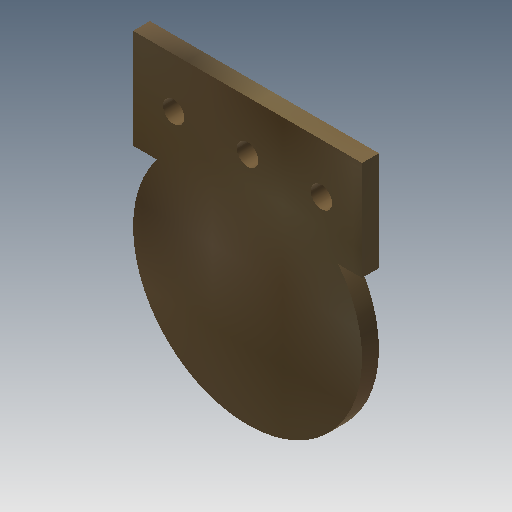
# Autodesk Inventor part: Part3_panel pot
Saved by Autodesk Inventor 2020 (Build 240168000, 168)
## iProperties
Created: 2016-08-22
Part Number: Part3_panel pot
Material: Generic
Document SubType Name: Modeling
Designer: Tom
Density: 1 g/cm^3
Appearance: Default
Author: Tom
Autodesk Inventor part; units mm, degrees
ref_plane "YZ Plane" through (0, 0, 0) normal (1, 0, 0) x (0, 1, 0)
ref_plane "XZ Plane" through (0, 0, 0) normal (0, 1, 0) x (-1, 0, 0)
ref_plane "XY Plane" through (0, 0, 0) normal (0, 0, 1) x (1, 0, 0)
sketch "Sketch1" plane through (0, 0, 0) normal (0, 0, 1) x (1, 0, 0)
  arc A0 (-6.1315, 4.735) -> (6.1315, 4.735) centre (0, 0) ccw
  line L0 (0, 0) -> (13.0157, 0) construction
  line L1 (7.747, 4.735) -> (7.747, 11.466)
  line L2 (7.747, 11.466) -> (-7.747, 11.466)
  line L3 (-7.747, 11.466) -> (-7.747, 4.735)
  line L4 (-7.747, 4.735) -> (-6.1315, 4.735)
  line L5 (6.1315, 4.735) -> (7.747, 4.735)
  dimension "d0" = 15.494
  dimension "d1" = 6.731
  dimension "d2" = 15.494
  dimension "d3" = 7.747
  constraints: 12 end point, 3 horizontal, 3 parallel, 2 perpendicular, 2 point on circle, 1 centre point, 1 coincident
  measures "d0" diameter of A0
  measures "d1" distance of L2.end L3.end
  measures "d2" distance of L1.end L2.end
  measures "d3" distance from line of L1 point (0, 0)
extrude "Extrusion1" add sketch "Sketch1" along normal blind 1.143
sketch "Sketch2" plane through (0, 0, 1.143) normal (0, 0, 1) x (1, 0, 0)
  line L0 (7.747, 11.466) -> (-7.747, 11.466) projected
  point P0 (-7.747, 4.735)
  point P1 (-5, 8.1005)
  point P2 (0, 8.1005)
  point P3 (5, 8.1005)
  dimension "d6" = 5
  dimension "d7" = 5
  dimension "d8" = 6.731
  dimension "d9" = 3.3655
  measures "d6" distance of point (-5, 8.101) point (0, 8.101)
  measures "d7" distance of point (0, 8.101) point (5, 8.101)
  measures "d8" distance of L0.end point (-7.747, 4.735)
  measures "d9" distance from line of L0 point (-5, 8.101)
hole "Hole1" at (-5, 8.1005, 1.143) at (0, 8.1005, 1.143) at (5, 8.1005, 1.143) direction (0, 0, -1) diameter 1.4478 end through all
equation "\"d3\" = 0.5 * d2"
equation "\"d9\" = 0.5 * d8"
body "Solid1"
